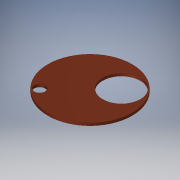
# Autodesk Inventor part: 2K8 stage mini
Saved by Autodesk Inventor 2018 (Build 220112000, 112)
## iProperties
Created: 2018-10-16
Part Number: 2K8 stage mini
Material: Copper
Document SubType Name: Modeling
Designer: freyja
Density: 8.94 g/cm^3
Appearance: Copper - Satin
Mass: 746.074 g
Surface Area: 976.476 cm^2
Volume: 276.324 cm^3
Author: freyja
Autodesk Inventor part; units mm, degrees
ref_plane "YZ Plane" through (0, 0, 0) normal (1, 0, 0) x (0, 1, 0)
ref_plane "XZ Plane" through (0, 0, 0) normal (0, 1, 0) x (-1, 0, 0)
ref_plane "XY Plane" through (0, 0, 0) normal (0, 0, 1) x (1, 0, 0)
sketch "Sketch2" plane through (0, 0, 0) normal (0, 1, 0) x (-1, 0, 0)
  line L0 (0, 0) -> (-24.2467, -24.2467) construction
  line L1 (0, 0) -> (-34.29, 0) construction
  circle A0 centre (-24.2467, -24.2467) radius 107.95
  dimension "d6" = 34.29
  dimension "d7" = 315
  dimension "d8" = 215.9
  constraints: 4 end point, 1 centre point, 1 coincident, 1 equal length, 1 horizontal
  measures "d6" distance of L0.start L0.end
  measures "d8" diameter of A0
extrude "Extrusion1" add sketch "Sketch2" against normal blind 6.35
sketch "Sketch1" plane through (0, 0, 0) normal (0, 1, 0) x (-1, 0, 0)
  line L0 (0, 0) -> (-64.6578, -64.6578) construction
  line L1 (0, 0) -> (91.44, 0) construction
  circle A0 centre (-64.6578, -64.6578) radius 48.26
  line L2 (0, 0) -> (40.4112, 40.4112) construction
  line L3 (0, 0) -> (57.15, 0) construction
  circle A1 centre (40.4112, 40.4112) radius 13.97
  dimension "d0" = 91.44
  dimension "d1" = 135
  dimension "d2" = 96.52
  dimension "d3" = 57.15
  dimension "d4" = 45
  dimension "d5" = 27.94
  constraints: 8 end point, 2 centre point, 2 coincident, 2 equal length, 2 horizontal
  measures "d0" distance of L0.start L0.end
  measures "d1" angle of L0 L1
  measures "d2" diameter of A0
  measures "d3" distance of L0.start L2.end
  measures "d4" angle of L3 L2
  measures "d5" diameter of A1
extrude "Extrusion2" cut sketch "Sketch1" against normal up to surface (6.35 mm away)
sketch "Sketch9" plane through (24.2467, 0, -24.2467) normal (0, 1, 0) x (1, 0, 0)
  circle A0 centre (40.4112, 40.4112) radius 48.26 projected
  circle A1 centre (-64.6578, -64.6578) radius 13.97 projected
  line L0 (40.4112, 40.4112) -> (-64.6578, -64.6578)
  circle A2 centre (-29.6348, -29.6348) radius 63.5
  circle A3 centre (29.6348, 29.6348) radius 63.5
  circle A4 centre (40.4112, 40.4112) radius 48.26 projected
  line L1 (-33.7328, 33.7328) -> (33.7328, -33.7328)
  point P0 (-24.2467, -24.2467)
  dimension "d81" = 127
  dimension "d82" = 127
  constraints: 4 end point, 4 point on circle, 2 centre point, 2 point on line, 2 tangent
  measures "d81" diameter of A2
  measures "d82" diameter of A3
body "Solid1"
